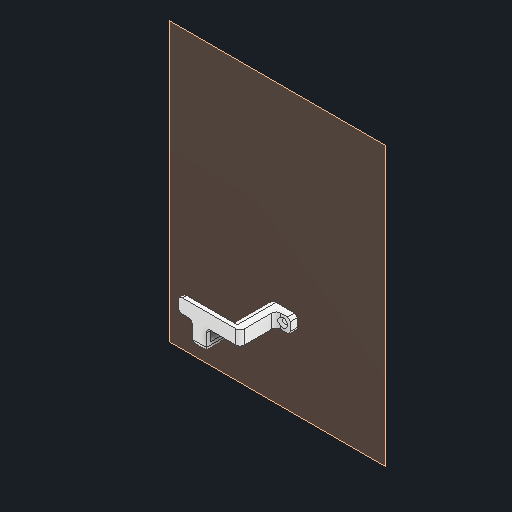
# Autodesk Inventor part: FrontBracket
Saved by Autodesk Inventor 2023 (Build 270158000, 158)
## iProperties
Created: 2023-09-27
Part Number: FrontBracket
Material: Пластик ПАЭК
Document SubType Name: Modeling
Designer: khrip
Density: 1.32 g/cm^3
Appearance: Гладкий — белый
Author: khrip
Autodesk Inventor part; units mm, degrees
ref_plane "YZ Plane" through (0, 0, 0) normal (1, 0, 0) x (0, 1, 0)
ref_plane "XZ Plane" through (0, 0, 0) normal (0, 1, 0) x (-1, 0, 0)
ref_plane "XY Plane" through (0, 0, 0) normal (0, 0, 1) x (1, 0, 0)
ref_plane "РабПлоскость1" through (0, 0, 0) normal (0, 0, 1) x (1, 0, 0)
sketch "Эскиз1" plane through (0, 0, 0) normal (0, 0, 1) x (1, 0, 0)
  line L0 (-6, -50.525) -> (-6, 46.475) projected
  arc A0 (-10, -54.525) -> (-6, -50.525) centre (-10, -50.525) ccw projected
  line L1 (-36, -54.525) -> (-10, -54.525) projected
  arc A1 (-40, -50.525) -> (-36, -54.525) centre (-36, -50.525) ccw projected
  line L2 (-40, 46.475) -> (-40, -50.525) projected
  circle A2 centre (-1, -39.525) radius 5
  line L3 (5, 13.475) -> (5, 17.5589) projected
  line L4 (14, -44.525) -> (4, -44.525)
  line L5 (4, -44.525) -> (4, -34.525)
  line L6 (4, -34.525) -> (14, -34.525)
  line L7 (14, -34.525) -> (14, -44.525)
  line L8 (4, -44.525) -> (-1, -44.525)
  line L9 (-1, -44.525) -> (-1, -34.525)
  line L10 (-1, -34.525) -> (4, -34.525)
  line L11 (4, -34.525) -> (4, -44.525)
  point P0 (0, 0)
  dimension "d0" = 10
  dimension "d1" = 10
  dimension "d2" = 5
  dimension "d3" = 10
  dimension "d4" = 15
  dimension "d5" = 20
  constraints: 16 end point, 4 parallel, 2 horizontal, 2 perpendicular, 1 midpoint, 1 vertical, 3 other
  measures "d1" distance of L5.end L6.end
  measures "d2" distance of L9.end L10.end
  measures "d3" distance between parallel lines of L1 L4
  measures "d4" distance from line of L1 point (-1, -39.525)
  measures "d5" distance between parallel lines of L6 L1
extrude "Выдавливание1" add sketch "Эскиз1" along normal blind 5
sketch "Эскиз2" plane through (0, 0, 5) normal (0, 0, 1) x (1, 0, 0)
  line L0 (-1, -44.525) -> (14, -44.525) projected
  line L1 (14, -44.525) -> (14, -34.525) projected
  line L2 (14, -34.525) -> (-1, -34.525) projected
  arc A0 (-1, -34.525) -> (-1, -44.525) centre (-1, -39.525) ccw projected
  circle A1 centre (-1, -39.525) radius 5
  line L3 (-1, -44.525) -> (4, -44.525)
  line L4 (4, -44.525) -> (4, -34.525)
  line L5 (4, -34.525) -> (-1, -34.525)
  line L6 (-1, -34.525) -> (-1, -44.525)
  point P0 (0, 0)
  point P1 (4, -44.525)
  dimension "d8" = 10
  constraints: 8 end point, 2 parallel, 1 coincident, 1 horizontal, 1 perpendicular, 1 point on line, 1 vertical alignment, 2 other
  measures "d8" distance between parallel lines of L1 L4
extrude "Выдавливание2" add sketch "Эскиз2" along normal blind 22.5 contours A1 L4 L0 | L6 A1 | A0 L6 | L2 L4 A1
sketch "Эскиз3" plane through (0, 0, 27.5) normal (0, 0, 1) x (1, 0, 0)
  line L0 (-1, -44.525) -> (4, -44.525) projected
  line L1 (4, -44.525) -> (4, -34.525) projected
  line L2 (4, -34.525) -> (-1, -34.525) projected
  arc A0 (-1, -34.525) -> (-1, -44.525) centre (-1, -39.525) ccw projected
  line L3 (4, -34.525) -> (-40, -34.525)
  line L4 (-40, -34.525) -> (-40, -44.525)
  line L5 (-40, -44.525) -> (4, -44.525)
  line L6 (4, -44.525) -> (4, -34.525)
  line L7 (-40, 46.475) -> (-40, -50.525) projected
  line L8 (-30, -34.525) -> (-20, -34.525)
  line L9 (-20, -34.525) -> (-20, -59.525)
  line L10 (-20, -59.525) -> (-30, -59.525)
  line L11 (-30, -59.525) -> (-30, -34.525)
  line L12 (-36, -54.525) -> (-10, -54.525) projected
  point P0 (0, 0)
  point P1 (-1, -34.525)
  point P2 (-20, -44.525)
  point P3 (-30, -44.525)
  dimension "d11" = 0
  dimension "d12" = 10
  dimension "d24" = 10
  dimension "d25" = 10
  dimension "d26" = 5
  constraints: 16 end point, 4 parallel, 2 horizontal, 2 perpendicular, 1 point on line
  measures "d11" distance between parallel lines of L7 L4
  measures "d12" distance between parallel lines of L3 L5
  measures "d24" distance of L9.end L10.end
  measures "d25" distance between parallel lines of L7 L11
  measures "d26" distance between parallel lines of L10 L12
extrude "Выдавливание3" add sketch "Эскиз3" along normal blind 3
sketch "Эскиз4" plane through (0, 0, 5) normal (0, 0, 1) x (1, 0, 0)
  line L0 (4, -34.525) -> (4, -44.525) projected
  line L1 (4, -44.525) -> (14, -44.525) projected
  line L2 (14, -44.525) -> (14, -34.525) projected
  line L3 (14, -34.525) -> (4, -34.525) projected
  circle A0 centre (9, -39.525) radius 1.6899
  point P0 (0, 0)
  constraints: 1 centre point
hole "Отверстие1" at (9, -39.525, 5) direction (0, 0, -1) diameter 3.4 end through all countersink diameter 6.3 countersink angle 90 clearance for "Винт с потайной головкой ISO 2009/7046" size "M3" standard "ISO"
fillet "Сопряжение1" radius 2 2 edges at (14, -34.525, 2.5) (14, -44.525, 2.5)
fillet "Сопряжение2" radius 3 2 edges at (4, -39.525, 5) (4, -39.525, 30.5)
sketch "Эскиз5" plane through (0, 0, 27.5) normal (0, 0, -1) x (-1, 0, 0)
  line L0 (30, -59.525) -> (20, -59.525) projected
  line L1 (30, -44.525) -> (30, -59.525) projected
  line L2 (20, -59.525) -> (30, -59.525)
  line L3 (30, -59.525) -> (30, -54.525)
  line L4 (30, -54.525) -> (20, -54.525)
  line L5 (20, -54.525) -> (20, -59.525)
  point P0 (0, 0)
  dimension "d27" = 5
  constraints: 8 end point, 2 parallel, 1 horizontal, 1 perpendicular, 1 point on line
  measures "d27" distance of L3.end L2.end
extrude "Выдавливание4" add sketch "Эскиз5" along normal blind 10
fillet "Сопряжение3" radius 3 8 edges at (-20, -44.525, 29) (-30, -44.525, 29) (-40, -44.525, 29) (-40, -34.525, 29) (-20, -59.525, 24) (-30, -59.525, 24) (-25, -59.525, 30.5) (-25, -59.525, 17.5)
